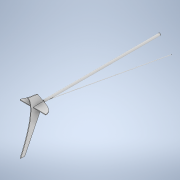
# Autodesk Inventor part: tail
Saved by Autodesk Inventor 2020 (Build 240168000, 168)
## iProperties
Created: 2019-06-11
Part Number: tail
Material: Generic
Document SubType Name: Modeling
Designer: Vivek Muskan
Density: 1 g/cm^3
Appearance: Default
Author: Vivek Muskan
Autodesk Inventor part; units mm, degrees
ref_plane "YZ Plane" through (0, 0, 0) normal (1, 0, 0) x (0, 1, 0)
ref_plane "XZ Plane" through (0, 0, 0) normal (0, 1, 0) x (-1, 0, 0)
ref_plane "XY Plane" through (0, 0, 0) normal (0, 0, 1) x (1, 0, 0)
sketch "Sketch1" plane through (0, 0, 0) normal (0, 0, 1) x (1, 0, 0)
  circle A0 centre (0, 0) radius 8.5
  circle A1 centre (0, 0) radius 7.5
  line L0 (0, 0) -> (91, 0)
  circle A2 centre (91, 0) radius 2
  line L1 (0, 0) -> (-91, 0)
  circle A3 centre (-91, 0) radius 2
  dimension "d0" = 17
  dimension "d1" = 15
  dimension "d2" = 91
  dimension "d3" = 4
  dimension "d4" = 91
  dimension "d5" = 4
  constraints: 4 centre point, 4 coincident, 4 end point, 2 horizontal
  measures "d0" diameter of A0
  measures "d1" diameter of A1
  measures "d2" distance of L0.start L0.end
  measures "d3" diameter of A2
  measures "d4" distance of L0.start L1.end
  measures "d5" diameter of A3
extrude "Extrusion1" add sketch "Sketch1" along normal blind 900 contours L0 A1 L1 A0 | A0 L1 A1 L0
sketch "Sketch2" plane through (0, 0, 900) normal (0, 0, 1) x (1, 0, 0)
  circle A0 centre (0, 0) radius 2
  dimension "d8" = 4
  constraints: 1 centre point, 1 coincident
  measures "d8" diameter of A0
sketch "Sketch3" plane through (0, 0, 0) normal (0, 0, -1) x (-1, 0, 0)
  line L0 (0, 0) -> (91, 0)
  line L1 (91, 0) -> (91, -91)
  circle A0 centre (91, -91) radius 2
  dimension "d9" = 91
  dimension "d11" = 91
  dimension "d12" = 4
  constraints: 4 end point, 1 centre point, 1 coincident, 1 horizontal, 1 vertical
  measures "d9" distance of L0.start L0.end
  measures "d11" distance of L0.end L1.end
  measures "d12" diameter of A0
loft "Loft1" add profiles "Sketch3", "Sketch2"
mirror "Mirror1" about plane through (0, 0, 0) normal (1, 0, 0) of "Loft1"
sketch "Sketch4" plane through (0, 0, 0) normal (0, 1, 0) x (-1, 0, 0)
  line L0 (0, 880.2198) -> (0, 900) projected
  line L1 (0, 880.2198) -> (0, 980.2198)
  line L2 (0, 980.2198) -> (100, 980.2198)
  line L3 (100, 980.2198) -> (100, 930.2198) construction
  line L4 (100, 930.2198) -> (0, 900) construction
  spline S0 degree 2 poles (100, 980.2198) (100, 930.2198) (0, 900) knots 1 1 1 2 2 2
  line L5 (0, 980.2198) -> (-100, 980.2198)
  line L6 (-100, 980.2198) -> (-100, 930.2198) construction
  line L7 (-100, 930.2198) -> (0, 900) construction
  spline S1 degree 2 poles (-100, 980.2198) (-100, 930.2198) (0, 900) knots 1 1 1 2 2 2
  point P0 (0, 0)
  dimension "d17" = 100
  dimension "d18" = 100
  constraints: 6 end point, 2 symmetric about line, 1 collinear, 1 perpendicular, 1 vertical, 6 other
  measures "d17" distance of L0.start L1.end
  measures "d18" distance of L1.end L2.end
extrude "Extrusion2" add sketch "Sketch4" along normal mid plane 5
sketch "Sketch5" plane through (0, 0, 0) normal (1, 0, 0) x (0, 1, 0)
  line L0 (-2, 900) -> (2, 900) projected
  line L1 (2, 900) -> (71.1918, 946.4774)
  line L2 (71.1918, 946.4774) -> (83.6853, 1020.7039)
  line L3 (83.6853, 1020.7039) -> (-15.9768, 953.7591) construction
  line L4 (-15.9768, 953.7591) -> (-292.5919, 1077.2925) construction
  spline S0 degree 2 poles (83.6853, 1020.7039) (-15.9768, 953.7591) (-292.5919, 1077.2925) knots 1 1 1 2 2 2
  line L5 (-292.5919, 1077.2925) -> (-292.5919, 1045.873)
  line L6 (-292.5919, 1045.873) -> (2, 900)
  point P0 (0, 0)
  constraints: 8 end point, 1 vertical, 3 other
extrude "Extrusion3" add sketch "Sketch5" along normal mid plane 5
body "Solid1"
